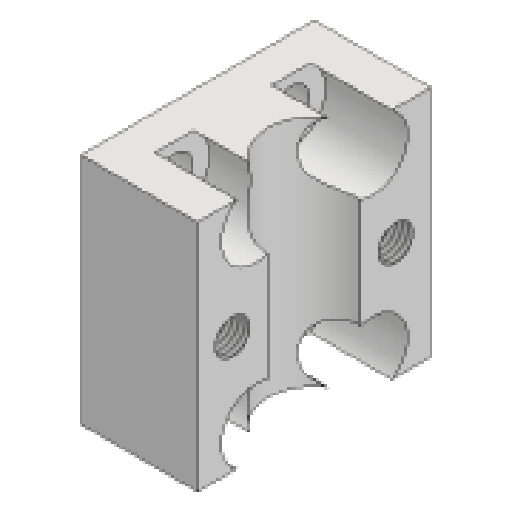
# Autodesk Inventor part: LinearClamp
Saved by Autodesk Inventor 2023 (Build 270158000, 158)
## iProperties
Created: 2022-10-30
Part Number: LinearClamp
Material: Generic
Document SubType Name: Modeling
Designer: deli
Density: 1 g/cm^3
Appearance: Default
Author: deli
Autodesk Inventor part; units mm, degrees
ref_plane "YZ Plane" through (0, 0, 0) normal (1, 0, 0) x (0, 1, 0)
ref_plane "XZ Plane" through (0, 0, 0) normal (0, 1, 0) x (-1, 0, 0)
ref_plane "XY Plane" through (0, 0, 0) normal (0, 0, 1) x (1, 0, 0)
sketch "Sketch2" plane through (0, 0, 0) normal (0, 1, 0) x (-1, 0, 0)
  line L0 (24.1917, -21.0916) -> (24.1917, -41.0916)
  line L1 (24.1917, -41.0916) -> (14.1917, -41.0916)
  line L2 (14.1917, -41.0916) -> (14.1917, -35.0916)
  line L3 (24.1917, -21.0916) -> (14.1917, -21.0916)
  line L4 (14.1917, -21.0916) -> (14.1917, -27.0916)
  arc A0 (14.1917, -35.0916) -> (14.1917, -27.0916) centre (14.1917, -31.0916) ccw
  point P0 (0, 0)
  dimension "d1" = 4
  dimension "d2" = 20
  dimension "d4" = 6
  constraints: 10 end point, 2 collinear, 2 perpendicular, 2 point on circle, 1 centre point, 1 horizontal, 1 parallel, 1 point on line, 1 vertical
  measures "d1" radius of A0
  measures "d2" distance of L0.start L0.end
  measures "d4" distance edge to line of A0 L0
extrude "Extrusion1" add sketch "Sketch2" along normal blind 20
sketch "Sketch3" plane through (-14.1917, 0, -21.0916) normal (1, 0, 0) x (0, 0, -1)
  circle A0 centre (5, 17.5) radius 1.6
  circle A1 centre (15, 17.5) radius 1.6
  line L0 (0, 0) -> (0, 20) projected
  line L1 (20, 0) -> (20, 20) projected
  circle A2 centre (5, 2.5) radius 1.6
  circle A3 centre (15, 2.5) radius 1.6
  line L2 (0, 20) -> (6, 20) projected
  line L3 (14, 20) -> (20, 20) projected
  point P0 (-21.0916, 0)
  dimension "d7" = 3.2
  dimension "d9" = 10
  dimension "d10" = 5
  dimension "d11" = 20
  dimension "d12" = 15
  dimension "d13" = 20
  dimension "d14" = 2.5
  dimension "d15" = 2.5
  dimension "d16" = 15
  dimension "d19" = 5
  dimension "d20" = 10
  constraints: 4 centre point, 3 equal radius
  measures "d7" diameter of A0
  measures "d9" distance of A1.centre A0.centre
  measures "d10" distance from line of L0 A0.centre
  measures "d11" distance between parallel lines of L0 L1
  measures "d12" distance of A2.centre A0.centre
  measures "d13" distance of L0.start L0.end
  measures "d14" distance from line of L2 A0.centre
  measures "d15" distance from line of L3 A1.centre
  measures "d16" distance of A1.centre A3.centre
  measures "d19" distance from line of L0 A2.centre
  measures "d20" distance of A3.centre A2.centre
extrude "Extrusion2" cut sketch "Sketch3" against normal blind 20
sketch "Sketch4" plane through (-14.1917, 0, -21.0916) normal (1, 0, 0) x (0, 0, -1)
  arc A0 (6, 18.749) -> (6, 16.251) centre (5, 17.5) ccw projected
  arc A1 (14, 16.251) -> (14, 18.749) centre (15, 17.5) ccw projected
  arc A2 (14, 1.251) -> (14, 3.749) centre (15, 2.5) ccw projected
  arc A3 (6, 3.749) -> (6, 1.251) centre (5, 2.5) ccw projected
  circle A4 centre (5, 17.5) radius 3
  circle A5 centre (15, 17.5) radius 3
  circle A6 centre (15, 2.5) radius 3
  circle A7 centre (5, 2.5) radius 3
  point P0 (-21.0916, 0)
  dimension "d21" = 6
  constraints: 4 centre point, 4 coincident, 3 equal radius
  measures "d21" diameter of A4
extrude "Extrusion3" cut sketch "Sketch4" against normal blind 8
sketch "Sketch5" plane through (-14.1917, 0, -21.0916) normal (1, 0, 0) x (0, 0, -1)
  circle A0 centre (2.4, 10) radius 1.5
  circle A1 centre (17.6, 10) radius 1.5
  line L0 (14, 5.3284) -> (14, 14.6716) projected
  line L1 (6, 5.3284) -> (6, 14.6716) projected
  line L2 (0, 0) -> (0, 20) projected
  line L3 (20, 0) -> (20, 20) projected
  point P0 (-21.0916, 0)
  dimension "d25" = 3
  dimension "d28" = 4.6716
  dimension "d29" = 9.3431
  dimension "d30" = 4.6716
  dimension "d37" = 2.4
  dimension "d38" = 2.4
  constraints: 2 centre point, 1 equal radius
  measures "d25" diameter of A1
  measures "d28" vertical distance of L1.end A0.centre
  measures "d29" distance of L1.start L1.end
  measures "d30" vertical distance of A1.centre L0.end
  measures "d37" distance from line of L2 A0.centre
  measures "d38" distance from line of L3 A1.centre
extrude "Extrusion4" cut sketch "Sketch5" against normal blind 8
thread "Thread1" size "M3x0.5" class "6H" standard "ANSI Metric M Profile" full length
thread "Thread2" size "M3x0.5" class "6H" standard "ANSI Metric M Profile" full length
equation "\"d10\" = -0.5 * d9 + 0.5 * d11"
equation "\"d14\" = -0.5 * d12 + 0.5 * d13"
equation "\"d15\" = d14"
equation "\"d16\" = d12"
equation "\"d19\" = d10"
equation "\"d20\" = d9"
equation "\"d28\" = 0.5 * d29"
equation "\"d30\" = d28"
equation "\"d38\" = d37"
body "Solid1"
